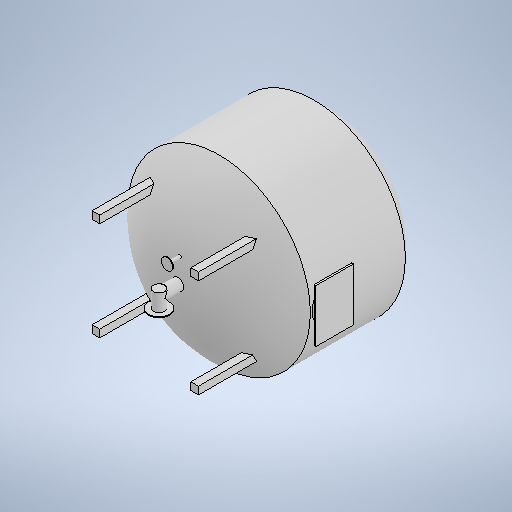
# Autodesk Inventor part: Фильтр контактный
Saved by Autodesk Inventor 2025 (Build 290162010, 162A)
## iProperties
Created: 2024-10-10
Part Number: Фильтр контактный
Material: Generic
Document SubType Name: Modeling
Designer: pokla
Density: 1 g/cm^3
Appearance: Default
Author: pokla
Autodesk Inventor part; units mm, degrees
ref_plane "YZ Plane" through (0, 0, 0) normal (1, 0, 0) x (0, 1, 0)
ref_plane "XY Plane" through (0, 0, 0) normal (0, 0, 1) x (1, 0, 0)
sketch "Sketch1" plane through (0, 0, 0) normal (0, 0, 1) x (1, 0, 0)
  line L0 (1200, -625) -> (1200, 625)
  line L1 (0, 1167) -> (0, -1167)
  arc A0 (0, -1167) -> (1200, -625) centre (45.2095, 332.3185) ccw
  arc A1 (1200, 625) -> (0, 1167) centre (45.2095, -332.3185) ccw
  point P0 (0, 0)
  point P1 (0, 0)
  dimension "d0" = 1250
  dimension "d1" = 542
  dimension "d2" = 542
  dimension "d3" = 2400
  dimension "d9" = 1500
  dimension "d10" = 1500
  constraints: 4 end point, 4 point on circle, 2 centre point, 2 vertical, 1 coincident, 1 midpoint
  measures "d0" distance of L0.start L0.end
  measures "d1" vertical distance of L0.end L1.start
  measures "d2" vertical distance of L0.start L1.end
  measures "d3" diameter of L0 L1
  measures "d9" radius of A0
  measures "d10" radius of A1
revolve "Revolution1" add sketch "Sketch1" angle 360 about axis through (0, 1167, 0) along (0, -1, 0)
sketch "Sketch2" plane through (0, 0, 0) normal (0, 1, 0) x (-1, 0, 0)
  line L0 (650, 650) -> (-650, 650) construction
  line L1 (-650, 650) -> (-650, -650) construction
  line L2 (-650, -650) -> (650, -650) construction
  line L3 (650, -650) -> (650, 650) construction
  line L4 (650, 650) -> (-650, -650) construction
  line L5 (700, 700) -> (600, 700)
  line L6 (600, 700) -> (600, 600)
  line L7 (600, 600) -> (700, 600)
  line L8 (700, 600) -> (700, 700)
  line L9 (700, 700) -> (600, 600)
  line L10 (700, -600) -> (600, -600)
  line L11 (600, -600) -> (600, -700)
  line L12 (600, -700) -> (700, -700)
  line L13 (700, -600) -> (600, -700)
  line L14 (700, -700) -> (700, -600)
  line L15 (-600, 700) -> (-700, 700)
  line L16 (-700, 700) -> (-700, 600)
  line L17 (-700, 600) -> (-600, 600)
  line L18 (-600, 700) -> (-700, 600)
  line L19 (-600, 600) -> (-600, 700)
  line L20 (-600, -600) -> (-700, -600)
  line L21 (-700, -600) -> (-700, -700)
  line L22 (-700, -700) -> (-600, -700)
  line L23 (-600, -600) -> (-700, -700)
  line L24 (-600, -700) -> (-600, -600)
  point P0 (0, 0)
  point P1 (0, 0)
  point P2 (650, -650)
  point P3 (0, -1300)
  point P4 (-650, 650)
  point P5 (-1300, 0)
  point P6 (-650, -650)
  point P7 (-1300, -1300)
  dimension "d12" = 1300
  dimension "d13" = 1300
  dimension "d16" = 100
  dimension "d17" = 100
  dimension "d24" = 1300
  dimension "d27" = 1300
  constraints: 50 end point, 4 parallel, 3 horizontal, 2 midpoint, 2 perpendicular, 1 coincident, 1 vertical, 33 other
  measures "d12" distance of L2.end L1.end
  measures "d13" distance of L0.end L1.end
  measures "d16" distance of L7.end L6.end
  measures "d17" distance of L6.end L5.end
  measures "d24" distance of L5.start L10.start
  measures "d27" distance of L5.start L15.start
extrude "Extrusion1" add sketch "Sketch2" against normal blind 1597
sketch "Sketch3" plane through (0, 0, 0) normal (0, 1, 0) x (-1, 0, 0)
  circle A0 centre (0, 0) radius 75
  dimension "d32" = 150
  constraints: 1 centre point, 1 coincident
  measures "d32" diameter of A0
extrude "Extrusion2" add sketch "Sketch3" along normal blind 1230
sketch "Sketch4" plane through (0, 1230, 0) normal (0, 1, 0) x (1, 0, 0)
  circle A0 centre (0, 0) radius 140
  dimension "d35" = 280
  constraints: 1 centre point, 1 coincident
  measures "d35" diameter of A0
extrude "Extrusion3" add sketch "Sketch4" along normal blind 12
sketch "Sketch5" plane through (0, 0, 0) normal (1, 0, 0) x (0, 1, 0)
  circle A0 centre (-378.75, 0) radius 225
  point P0 (0, 0)
  dimension "d38" = 378.75
  dimension "d39" = 450
  constraints: 1 centre point, 1 horizontal alignment
  measures "d38" distance of A0.centre point (0, 0)
  measures "d39" diameter of A0
extrude "Extrusion4" add sketch "Sketch5" along normal blind 1250
sketch "Sketch6" plane through (1250, -378.75, 0) normal (1, 0, 0) x (0, 0, -1)
  circle A0 centre (0, 0) radius 225 projected
  line L0 (-347.5, 247.5) -> (347.5, 247.5)
  line L1 (347.5, 247.5) -> (347.5, -247.5)
  line L2 (347.5, -247.5) -> (-347.5, -247.5)
  line L3 (-347.5, -247.5) -> (-347.5, 247.5)
  line L4 (-347.5, 247.5) -> (347.5, -247.5) construction
  point P0 (0, 378.75)
  dimension "d42" = 695
  dimension "d43" = 495
  constraints: 10 end point, 2 parallel, 1 coincident, 1 horizontal, 1 midpoint, 1 perpendicular
  measures "d42" distance of L1.end L2.end
  measures "d43" distance of L0.end L1.end
extrude "Extrusion5" add sketch "Sketch6" along normal blind 24 contours A0 | L0 L1 L2 L3
sketch "Sketch7" plane through (0, 0, 0) normal (0, 1, 0) x (-1, 0, 0)
  circle A0 centre (0, 0) radius 75
  dimension "d46" = 150
  constraints: 1 centre point, 1 coincident
  measures "d46" diameter of A0
extrude "Extrusion6" add sketch "Sketch7" against normal blind 1417
sketch "Sketch8" plane through (0, 0, 0) normal (0, 0, 1) x (1, 0, 0)
  line L0 (-75, -1417) -> (75, -1417) projected
  circle A0 centre (0, -1417) radius 75
  point P0 (0, 0)
  constraints: 1 horizontal alignment, 1 midpoint, 2 other
extrude "Extrusion7" add sketch "Sketch8" along normal blind 75 and the other way blind 150
sketch "Sketch9" plane through (0, -1417, -150) normal (0, 0, -1) x (-1, 0, 0)
  circle A0 centre (0, 0) radius 75 projected
  circle A1 centre (0, 0) radius 140
  point P0 (0, 1417)
  dimension "d53" = 280
  constraints: 1 centre point, 1 coincident
  measures "d53" diameter of A1
extrude "Extrusion8" add sketch "Sketch9" along normal blind 12 contours A0 | A1
sketch "Sketch10" plane through (0, 0, 0) normal (0, 1, 0) x (-1, 0, 0)
  circle A0 centre (0, 300) radius 20
  point P0 (0, 0)
  dimension "d56" = 40
  dimension "d57" = 300
  constraints: 1 centre point, 1 vertical alignment
  measures "d56" diameter of A0
  measures "d57" distance of point (0, 0) A0.centre
extrude "Extrusion9" add sketch "Sketch10" against normal blind 1300
sketch "Sketch11" plane through (0, -1300, 300) normal (0, -1, 0) x (1, 0, 0)
  circle A0 centre (0, 0) radius 20 projected
  circle A1 centre (0, 0) radius 75
  point P0 (0, -300)
  dimension "d60" = 150
  constraints: 1 centre point, 1 coincident
  measures "d60" diameter of A1
extrude "Extrusion10" add sketch "Sketch11" along normal blind 12 contours A0 | A1
sketch "Sketch12" plane through (0, 0, 0) normal (0, 0, 1) x (1, 0, 0)
  circle A0 centre (0, 513) radius 75
  point P0 (0, 0)
  dimension "d63" = 150
  dimension "d64" = 513
  constraints: 1 centre point, 1 vertical alignment
  measures "d63" diameter of A0
  measures "d64" distance of A0.centre point (0, 0)
extrude "Extrusion11" add sketch "Sketch12" against normal blind 1450
ref_plane "Work Plane1" through (0, 513, 0) normal (0, 1, 0) x (-1, 0, 0)
sketch "Sketch13" plane through (0, 513, 0) normal (0, 1, 0) x (-1, 0, 0)
  circle A0 centre (0, -1375) radius 75
  line L0 (-75, -1450) -> (75, -1450) projected
  point P0 (0, 0)
  point P1 (0, -1450)
  dimension "d68" = 150
  dimension "d81" = 75
  constraints: 1 centre point, 1 midpoint, 1 vertical alignment
  measures "d68" diameter of A0
  measures "d81" distance of point (0, -1450) A0.centre
extrude "Extrusion12" add sketch "Sketch13" against normal blind 150
sketch "Sketch15" plane through (0, 363, -1375) normal (0, -1, 0) x (-1, 0, 0)
  circle A0 centre (0, 0) radius 75 projected
  circle A1 centre (0, 0) radius 140
  point P0 (0, -1375)
  dimension "d75" = 280
  constraints: 1 centre point, 1 coincident
  measures "d75" diameter of A1
extrude "Extrusion14" add sketch "Sketch15" along normal blind 12 contours A0 | A1
equation "\"d2\" = d1"
equation "\"d13\" = d12"
body "Solid1"
